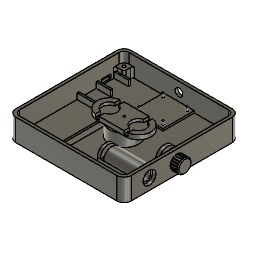
Microstir V2 (Autodesk Fusion 360 archive; units mm, degrees)
design "microstir" references "Type-C Lithium Battery Charger Board", "R300C DC Motor", "523450 Li-Ion Battery 3.7V 1000mAh", "PTFE Magnetic Stirrer Bar", "PWM DC motor speed controller", "Hexagon Socket Head Cap Screw STN EN ISO 4762 - M3 x 20 Steel 4.6 Plain"
Autodesk Fusion 360 part; units mm, degrees
(part 1 of 2)
sketch "Sketch1" plane through (0, 0, 0) normal (0, 0, 1) x (1, 0, 0)
  circle A0 centre (52.942, -52.6191) radius 1.6
  arc A1 (-47.558, -50.1191) -> (-49.558, -48.1191) centre (-49.558, -50.1191) ccw
  circle A2 centre (-52.058, -52.6191) radius 1.6
  line L0 (-49.558, -48.1191) -> (-54.558, -48.1191)
  arc A3 (-49.558, 47.8809) -> (-47.558, 49.8809) centre (-49.558, 49.8809) ccw
  line L1 (-56.558, -46.1191) -> (-56.558, 45.8809)
  line L2 (-59.558, -52.6191) -> (-59.558, 52.3809)
  arc A4 (-59.558, 52.3809) -> (-52.058, 59.8809) centre (-52.058, 52.3809) cw
  arc A5 (46.442, 56.8809) -> (48.442, 54.8809) centre (46.442, 54.8809) cw
  arc A6 (-45.558, -57.1191) -> (-47.558, -55.1191) centre (-45.558, -55.1191) cw
  line L3 (52.942, -60.1191) -> (-52.058, -60.1191)
  line L4 (-52.058, 59.8809) -> (52.942, 59.8809)
  arc A7 (-56.558, 45.8809) -> (-54.558, 47.8809) centre (-54.558, 45.8809) cw
  arc A8 (50.442, -48.1191) -> (48.442, -50.1191) centre (50.442, -50.1191) ccw
  arc A9 (48.442, 49.8809) -> (50.442, 47.8809) centre (50.442, 49.8809) ccw
  line L5 (48.442, 54.8809) -> (48.442, 49.8809)
  circle A10 centre (52.942, 52.3809) radius 1.6
  arc A11 (55.442, 47.8809) -> (57.442, 45.8809) centre (55.442, 45.8809) cw
  circle A12 centre (-52.058, 52.3809) radius 1.6
  arc A13 (-52.058, -60.1191) -> (-59.558, -52.6191) centre (-52.058, -52.6191) cw
  arc A14 (-47.558, 54.8809) -> (-45.558, 56.8809) centre (-45.558, 54.8809) cw
  line L6 (48.442, -50.1191) -> (48.442, -55.1191)
  arc A15 (-54.558, -48.1191) -> (-56.558, -46.1191) centre (-54.558, -46.1191) cw
  line L7 (57.442, 45.8809) -> (57.442, -46.1191)
  arc A16 (52.942, 59.8809) -> (60.442, 52.3809) centre (52.942, 52.3809) cw
  line L8 (50.442, 47.8809) -> (55.442, 47.8809)
  line L9 (-54.558, 47.8809) -> (-49.558, 47.8809)
  line L10 (55.442, -48.1191) -> (50.442, -48.1191)
  line L11 (60.442, 52.3809) -> (60.442, -52.6191)
  arc A17 (48.442, -55.1191) -> (46.442, -57.1191) centre (46.442, -55.1191) cw
  line L12 (-47.558, 49.8809) -> (-47.558, 54.8809)
  line L13 (-45.558, 56.8809) -> (46.442, 56.8809)
  line L14 (-47.558, -55.1191) -> (-47.558, -50.1191)
  arc A18 (57.442, -46.1191) -> (55.442, -48.1191) centre (55.442, -46.1191) cw
  arc A19 (60.442, -52.6191) -> (52.942, -60.1191) centre (52.942, -52.6191) cw
  line L15 (46.442, -57.1191) -> (-45.558, -57.1191)
  line L16 (-51.358, 56.8809) -> (52.242, 56.8809)
  line L17 (57.442, 51.6809) -> (57.442, -51.9191)
  line L18 (52.242, -57.1191) -> (-51.358, -57.1191)
  line L19 (-56.558, -51.9191) -> (-56.558, 51.6809)
  arc A20 (-51.358, 56.8809) -> (-56.558, 51.6809) centre (-51.358, 51.6809) ccw
  arc A21 (-56.558, -51.9191) -> (-51.358, -57.1191) centre (-51.358, -51.9191) ccw
  arc A22 (52.242, -57.1191) -> (57.442, -51.9191) centre (52.242, -51.9191) ccw
  arc A23 (57.442, 51.6809) -> (52.242, 56.8809) centre (52.242, 51.6809) ccw
  arc A24 (-79.7517, 57.5053) -> (-72.2517, 50.0053) centre (-79.7517, 50.0053) cw
  circle A25 centre (-79.7517, -54.9947) radius 1.6
  arc A26 (-184.7517, -62.4947) -> (-192.2517, -54.9947) centre (-184.7517, -54.9947) cw
  circle A27 centre (-184.7517, -54.9947) radius 1.6
  arc A28 (-72.2517, -54.9947) -> (-79.7517, -62.4947) centre (-79.7517, -54.9947) cw
  circle A29 centre (-184.7517, 50.0053) radius 1.6
  arc A30 (-192.2517, 50.0053) -> (-184.7517, 57.5053) centre (-184.7517, 50.0053) cw
  line L20 (-192.2517, -54.9947) -> (-192.2517, 50.0053)
  line L21 (-79.7517, -62.4947) -> (-184.7517, -62.4947)
  line L22 (-184.7517, 57.5053) -> (-79.7517, 57.5053)
  circle A31 centre (-79.7517, 50.0053) radius 1.6
  line L23 (-72.2517, 50.0053) -> (-72.2517, -54.9947)
  line L24 (-178.7517, 54.0053) -> (-85.7517, 54.0053)
  line L25 (-75.7517, 44.0053) -> (-75.7517, -48.9947)
  line L26 (-85.7517, -58.9947) -> (-178.7517, -58.9947)
  line L27 (-188.7517, -48.9947) -> (-188.7517, 44.0053)
  line L28 (-182.7517, -58.9947) -> (-184.2517, -58.9947)
  line L29 (-188.7517, -54.4947) -> (-188.7517, -52.9947)
  arc A32 (-80.2517, -58.9947) -> (-75.7517, -54.4947) centre (-80.2517, -54.4947) ccw
  arc A33 (-188.7517, -54.4947) -> (-184.2517, -58.9947) centre (-184.2517, -54.4947) ccw
  arc A34 (-184.2517, 54.0053) -> (-188.7517, 49.5053) centre (-184.2517, 49.5053) ccw
  line L30 (-132.2517, 54.0053) -> (-132.2517, -58.9947)
  line L31 (0.442, 56.8809) -> (0.442, -57.1191)
  line L32 (-75.7517, -52.9947) -> (-75.7517, -54.4947)
  line L33 (-81.7517, -58.9947) -> (-80.2517, -58.9947)
  line L34 (-75.7517, -48.9947) -> (-75.7517, -52.9947)
  line L35 (-85.7517, 54.0053) -> (-80.2517, 54.0053)
  line L36 (-184.2517, 54.0053) -> (-178.7517, 54.0053)
  line L37 (-188.7517, 44.0053) -> (-188.7517, 49.5053)
  line L38 (-188.7517, -48.9947) -> (-188.7517, -51)
  line L39 (-188.7517, -51) -> (-188.7517, -52.9947)
  line L40 (-178.7517, -58.9947) -> (-182.7517, -58.9947)
  line L41 (-85.7517, -58.9947) -> (-81.7517, -58.9947)
  line L42 (-74.6605, -54.9947) -> (-79.7517, -49.9035)
  line L43 (-79.7517, -49.9035) -> (-84.8428, -54.9947)
  line L44 (-84.8428, -54.9947) -> (-79.7517, -60.0858)
  line L45 (-79.7517, -60.0858) -> (-74.6605, -54.9947)
  line L46 (-74.6605, -54.9947) -> (-84.8428, -54.9947) construction
  line L47 (-79.7517, -49.9035) -> (-79.7517, -60.0858) construction
  line L48 (-84.8428, -54.9947) -> (-86.8428, -54.9947)
  line L49 (-86.8428, -54.9947) -> (-83.7517, -58.0858)
  line L50 (-79.7517, -49.9035) -> (-79.7517, -47.9035)
  line L51 (-79.7517, -47.9035) -> (-76.6605, -50.9947)
  line L52 (-76.6605, -50.9947) -> (-75.7517, -52.9947)
  line L53 (-83.7517, -58.0858) -> (-81.7517, -58.9947)
  line L54 (-79.7517, -47.9035) -> (-86.8428, -54.9947)
  line L55 (-79.7517, 44.9142) -> (-74.6605, 50.0053)
  line L56 (-74.6605, 50.0053) -> (-79.7517, 55.0965)
  line L57 (-79.7517, 55.0965) -> (-84.8428, 50.0053)
  line L58 (-84.8428, 50.0053) -> (-79.7517, 44.9142)
  line L59 (-84.8428, 50.0053) -> (-86.8428, 50.0053)
  line L60 (-86.8428, 50.0053) -> (-79.7517, 42.9142)
  line L61 (-86.8428, 50.0053) -> (-83.7517, 53.0965)
  line L62 (-83.7517, 53.0965) -> (-81.7517, 54.0053)
  line L63 (-81.7517, 54.0053) -> (-80.2517, 54.0053)
  line L64 (-75.7517, 48.0053) -> (-75.7517, 49.5053)
  arc A35 (-75.7517, 49.5053) -> (-80.2517, 54.0053) centre (-80.2517, 49.5053) ccw
  line L65 (-76.6605, 46.0053) -> (-75.7517, 48.0053)
  line L66 (-79.7517, 42.9142) -> (-76.6605, 46.0053)
  line L67 (-79.7517, 44.9142) -> (-79.7517, 42.9142)
  circle A36 centre (-79.7517, 50.0053) radius 1.6
  line L68 (-75.7517, 44.0053) -> (-75.7517, 48.7553)
  line L69 (-177.6605, -54.9947) -> (-184.7517, -47.9035)
  line L70 (-184.7517, -49.9035) -> (-184.7517, -47.9035)
  line L71 (-189.8428, -54.9947) -> (-184.7517, -60.0858)
  line L72 (-184.7517, -60.0858) -> (-179.6605, -54.9947)
  line L73 (-184.7517, -49.9035) -> (-189.8428, -54.9947)
  line L74 (-187.8428, -50.9947) -> (-188.7517, -52.9947)
  line L75 (-184.7517, -47.9035) -> (-187.8428, -50.9947)
  line L76 (-188.7517, -52.9947) -> (-188.7517, -54.4947)
  line L77 (-182.7517, -58.9947) -> (-184.2517, -58.9947)
  arc A37 (-188.7517, -54.4947) -> (-184.2517, -58.9947) centre (-184.2517, -54.4947) ccw
  line L78 (-180.7517, -58.0858) -> (-182.7517, -58.9947)
  line L79 (-177.6605, -54.9947) -> (-180.7517, -58.0858)
  line L80 (-179.6605, -54.9947) -> (-177.6605, -54.9947)
  line L81 (-179.6605, -54.9947) -> (-184.7517, -49.9035)
  circle A38 centre (-184.7517, -54.9947) radius 1.6
  line L82 (-184.7517, 42.9142) -> (-177.6605, 50.0053)
  line L83 (-184.7517, 44.9142) -> (-179.6605, 50.0053)
  line L84 (-184.7517, 55.0965) -> (-189.8428, 50.0053)
  line L85 (-189.8428, 50.0053) -> (-184.7517, 44.9142)
  line L86 (-179.6605, 50.0053) -> (-184.7517, 55.0965)
  line L87 (-179.6605, 50.0053) -> (-177.6605, 50.0053)
  line L88 (-180.7517, 53.0965) -> (-182.7517, 54.0053)
  line L89 (-182.7517, 54.0053) -> (-184.2517, 54.0053)
  arc A39 (-184.2517, 54.0053) -> (-188.7517, 49.5053) centre (-184.2517, 49.5053) ccw
  line L90 (-188.7517, 48.0053) -> (-188.7517, 49.5053)
  line L91 (-187.8428, 46.0053) -> (-188.7517, 48.0053)
  line L92 (-184.7517, 42.9142) -> (-187.8428, 46.0053)
  line L93 (-177.6605, 50.0053) -> (-180.7517, 53.0965)
  line L94 (-184.7517, 44.9142) -> (-184.7517, 42.9142)
  circle A40 centre (-184.7517, 50.0053) radius 1.6
  point P0 (52.942, -52.6191)
  point P1 (0.442, -0.1191)
  point P2 (-52.058, -52.6191)
  point P3 (-52.058, 52.3809)
  point P4 (52.942, 52.3809)
  point P5 (-79.7517, -54.9947)
  point P6 (-184.7517, -54.9947)
  point P7 (-184.7517, 50.0053)
  point P8 (-79.7517, 50.0053)
  point P9 (-132.2517, -2.4947)
  point P10 (-79.7517, -54.9947)
  point P11 (-79.7517, -54.9947)
  dimension "d1" = 5.2
  dimension "d195" = 7.2
  dimension "d196" = 7.2
  dimension "d199" = 2
  dimension "d202" = 2
  dimension "d203" = 7.2
  dimension "d204" = 7.2
  dimension "d205" = 2
  dimension "d206" = 2
  dimension "d207" = 7.2
  dimension "d208" = 7.2
  dimension "d209" = 2
  dimension "d210" = 2
  dimension "d211" = 7.2
  dimension "d212" = 7.2
  dimension "d213" = 2
  dimension "d214" = 2
  constraint horizontal L16
  constraint vertical L17
  constraint horizontal L18
  constraint vertical L19
  constraint tangent L16 A20
  constraint tangent L19 A20
  constraint tangent L18 A21
  constraint tangent L19 A21
  constraint equal A20 A21
  constraint tangent L17 A22
  constraint tangent L18 A22
  constraint equal A20 A22
  constraint tangent L16 A23
  constraint tangent L17 A23
  constraint equal A20 A23
  constraint horizontal L24
  constraint perpendicular L24 L25
  constraint parallel L24 L26
  constraint parallel L25 L27
  constraint coincident P11 P10
  constraint horizontal L28
  constraint vertical L29
  constraint tangent L28 A32
  constraint tangent L28 A33
  constraint tangent L29 A33
  constraint tangent L29 A34
  constraint midpoint L24 L30.start
  constraint midpoint L26 L30.end
  constraint midpoint L13 L31.start
  constraint midpoint L15 L31.end
  constraint coincident L28 A32.start
  constraint coincident L29 A34.end
  constraint coincident L25.end L32
  constraint coincident L26.start L33
  constraint perpendicular L42 L43
  constraint parallel L42 L44
  constraint parallel L43 L45
  constraint coincident L46 P11
  constraint coincident L47 P11
  constraint parallel L46 L48
  constraint vertical L50
  constraint perpendicular L49 L54
  constraint perpendicular L57 L58
  constraint parallel L55 L57
  constraint parallel L56 L58
  constraint perpendicular L60 L66
  constraint midpoint L64 L68.end
  constraint parallel L64 L68
  constraint perpendicular L72 L81
  constraint parallel L72 L73
  constraint parallel L71 L81
  constraint perpendicular L69 L75
  constraint perpendicular L83 L85
  constraint parallel L85 L86
  constraint parallel L83 L84
  constraint perpendicular L82 L93
  measures "d1" radius of A20
  measures "d195" distance of L43.end L44.end
  measures "d196" distance of L42.end L43.end
  measures "d199" distance of L43.end L48.end
  measures "d202" distance of L42.end L50.end
  measures "d203" distance of L55.end L55.start
  measures "d204" distance of L57.end L55.start
  measures "d205" distance of L55.start L60.end
  measures "d206" distance of L57.end L59.end
  measures "d207" distance of L71.start L70.start
  measures "d208" distance of L72.end L70.start
  measures "d209" distance of L70.start L69.end
  measures "d210" distance of L72.end L69.start
  measures "d211" distance of L84.start L83.end
  measures "d212" distance of L83.start L83.end
  measures "d213" distance of L82.end L83.end
  measures "d214" distance of L83.start L82.start
extrude "Extrude1" add sketch "Sketch1" along normal blind 2 contours A24 A26 A28 A30 L20 L21 L22 L23 | A25 | A27 A38 | A29 A40 | A31 A36 | L24 L26 L27 L30 L36 L37 L38 L39 L40 L69 L74 L75 L78 L79 L82 L88 L91 L92 L93 | L24 L25 L26 L30 L34 L35 L41 L49 L51 L52 L53 L54 L60 L61 L62 L65 L66 L68 | L36 L86 L87 L88 L89 L93 | A34 L36 L37 L83 L84 L85 L86 L89 A39 L90 | A34 L36 L84 L86 L89 A39 | L35 L57 L59 L61 L62 L63 | L82 L83 L87 L94 | L35 L56 L57 L63 A35 | L35 L55 L56 L57 L58 L63 L64 A35 | L33 L44 L48 L49 L53 | L28 L72 L77 L78 L79 L80 | A34 L84 A39 | L37 L85 L90 L91 L92 L94 | L58 L59 L60 L67 | A32 L32 L33 L42 L43 L44 L45 | A32 L33 L44 L45 | L28 A33 L71 L72 L77 A37 | L28 L29 A33 L71 L72 L73 L76 L77 A37 L81 | A34 L37 L84 L85 A39 L90 | L56 A35 | L55 L64 L65 L66 L67 L68 | L43 L48 L50 L54 | L69 L70 L80 L81 | L55 L56 L64 A35 | A32 L45 | L32 L42 L50 L51 L52 | A33 L71 A37 | L29 L70 L73 L74 L75 L76 | A32 L32 L42 L45 | L29 A33 L71 L73 L76 A37 makes body 1
extrude "Extrude2" add sketch "Sketch1" along normal blind 2.5 separate body contours A1 L0 A3 L1 A6 A7 A14 A15 L9 L12 L13 L14 L15 L16 L18 L19 L31 | A5 A8 A9 L5 A11 L6 L7 L8 L10 A17 L13 A18 L15 L16 L17 L18 L31 makes body 2
extrude "Extrude3" add sketch "Sketch1" along normal blind 23 contours L2 A4 L3 L4 A13 A16 L11 A19 bodies 2
extrude "Extrude20" add sketch "Sketch1" along normal blind 10 from surface at 2 contours L36 L86 L87 L88 L89 L93 | A34 L36 L37 L83 L84 L85 L86 L89 A39 L90 | L35 L57 L59 L61 L62 L63 | L82 L83 L87 L94 | L35 L55 L56 L57 L58 L63 L64 A35 | L33 L44 L48 L49 L53 | L28 L72 L77 L78 L79 L80 | A34 L84 A39 | L37 L85 L90 L91 L92 L94 | L58 L59 L60 L67 | A32 L32 L33 L42 L43 L44 L45 | L28 L29 A33 L71 L72 L73 L76 L77 A37 L81 | L56 A35 | L55 L64 L65 L66 L67 L68 | L43 L48 L50 L54 | L69 L70 L80 L81 | A32 L45 | L32 L42 L50 L51 L52 | A33 L71 A37 | L29 L70 L73 L74 L75 L76 bodies 1
extrude "Extrude21" add sketch "Sketch1" along normal blind 12.5 contours A1 L0 A6 A15 L14 L18 L19 A21 | A3 A7 A14 L9 L12 L16 L19 A20 | A8 L6 L10 A17 A18 L17 L18 A22 | A5 A9 L5 A11 L8 L16 L17 A23 bodies 2
sketch "Sketch12" plane through (0, 0, 12) normal (0, 0, 1) x (-1, 0, 0)
  line L0 (81.7517, 58.9947) -> (80.2517, 58.9947)
  arc A0 (80.2517, 58.9947) -> (75.7517, 54.4947) centre (80.2517, 54.4947) ccw
  line L1 (75.7517, 54.4947) -> (75.7517, 52.9947)
  circle A1 centre (79.7517, 54.9947) radius 3.1
  line L2 (79.7517, 59.3787) -> (79.7517, 50.6106) construction
  line L3 (84.1357, 54.9947) -> (75.3676, 54.9947) construction
  line L4 (79.7517, 49.9035) -> (84.8428, 54.9947)
  line L5 (84.8428, 54.9947) -> (79.7517, 60.0858)
  line L6 (79.7517, 60.0858) -> (74.6605, 54.9947)
  line L7 (74.6605, 54.9947) -> (79.7517, 49.9035)
  line L8 (79.7517, 49.9035) -> (79.7517, 60.0858) construction
  line L9 (84.8428, 54.9947) -> (74.6605, 54.9947) construction
  line L10 (79.7517, 60.0858) -> (74.6605, 60.0858)
  line L11 (74.6605, 60.0858) -> (74.6605, 54.9947)
  line L12 (74.6605, 54.9947) -> (79.7517, 54.9947)
  line L13 (79.7517, 54.9947) -> (79.7517, 60.0858)
  circle A2 centre (79.7517, 54.9947) radius 1.6
  line L14 (76.6605, 50.9947) -> (79.7517, 47.9035)
  line L15 (79.7517, 47.9035) -> (86.8428, 54.9947)
  line L16 (86.8428, 54.9947) -> (83.7517, 58.0858)
  line L17 (83.7517, 58.0858) -> (81.7517, 58.9947)
  line L18 (75.7517, 52.9947) -> (76.6605, 50.9947)
  line L19 (184.7517, 54.9947) -> (189.8428, 54.9947)
  line L20 (184.7517, 50.6106) -> (184.7517, 59.3787) construction
  circle A3 centre (184.7517, 54.9947) radius 3.1
  line L21 (189.8428, 60.0858) -> (184.7517, 60.0858)
  line L22 (179.6605, 54.9947) -> (184.7517, 49.9035)
  line L23 (184.7517, 49.9035) -> (189.8428, 54.9947)
  line L24 (184.7517, 49.9035) -> (184.7517, 60.0858) construction
  line L25 (189.8428, 54.9947) -> (189.8428, 60.0858)
  line L26 (184.7517, 60.0858) -> (179.6605, 54.9947)
  line L27 (189.8428, 54.9947) -> (184.7517, 60.0858)
  line L28 (189.1357, 54.9947) -> (180.3676, 54.9947) construction
  line L29 (179.6605, 54.9947) -> (189.8428, 54.9947) construction
  line L30 (184.7517, 60.0858) -> (184.7517, 54.9947)
  line L31 (79.7517, -55.0965) -> (79.7517, -50.0053)
  circle A4 centre (184.7517, -50.0053) radius 3.1
  line L32 (79.7517, -44.9142) -> (79.7517, -55.0965) construction
  line L33 (184.7517, -55.0965) -> (189.8428, -55.0965)
  line L34 (189.8428, -55.0965) -> (189.8428, -50.0053)
  line L35 (74.6605, -50.0053) -> (79.7517, -55.0965)
  line L36 (180.3676, -50.0053) -> (189.1357, -50.0053) construction
  line L37 (179.6605, -50.0053) -> (189.8428, -50.0053) construction
  line L38 (189.8428, -50.0053) -> (184.7517, -44.9142)
  line L39 (184.7517, -44.9142) -> (184.7517, -55.0965) construction
  line L40 (184.7517, -50.0053) -> (184.7517, -55.0965)
  line L41 (184.7517, -55.0965) -> (189.8428, -50.0053)
  line L42 (79.7517, -45.6213) -> (79.7517, -54.3894) construction
  line L43 (79.7517, -50.0053) -> (74.6605, -50.0053)
  line L44 (189.8428, -50.0053) -> (184.7517, -50.0053)
  line L45 (179.6605, -50.0053) -> (184.7517, -55.0965)
  line L46 (184.7517, -44.9142) -> (179.6605, -50.0053)
  circle A5 centre (79.7517, -50.0053) radius 3.1
  line L47 (79.7517, -55.0965) -> (84.8428, -50.0053)
  line L48 (84.8428, -50.0053) -> (74.6605, -50.0053) construction
  line L49 (74.6605, -50.0053) -> (74.6605, -55.0965)
  line L50 (75.3676, -50.0053) -> (84.1357, -50.0053) construction
  line L51 (74.6605, -55.0965) -> (79.7517, -55.0965)
  line L52 (84.8428, -50.0053) -> (79.7517, -44.9142)
  line L53 (79.7517, -44.9142) -> (74.6605, -50.0053)
  line L54 (184.7517, -54.3894) -> (184.7517, -45.6213) construction
  point P0 (79.7517, 54.9947)
  point P1 (79.7517, 54.9947)
  point P2 (184.7517, 54.9947)
  point P3 (184.7517, 54.9947)
  point P4 (79.7517, -50.0053)
  point P5 (79.7517, -50.0053)
  point P6 (184.7517, -50.0053)
  point P7 (184.7517, -50.0053)
  dimension "d184" = 6.2
  dimension "d190" = 7.2
  dimension "d191" = 7.2
  dimension "d215" = 6.2
  dimension "d216" = 7.2
  dimension "d217" = 7.2
  dimension "d218" = 6.2
  dimension "d219" = 7.2
  dimension "d220" = 7.2
  dimension "d221" = 6.2
  dimension "d222" = 7.2
  dimension "d223" = 7.2
  constraint coincident L2 P1
  constraint coincident L3 P1
  constraint coincident P1 P0
  constraint perpendicular L4 L5
  constraint parallel L4 L6
  constraint parallel L5 L7
  constraint coincident L8 P1
  constraint coincident L9 P1
  constraint horizontal L10
  constraint vertical L11
  constraint horizontal L12
  constraint vertical L13
  constraint coincident P3 L28
  constraint coincident P3 L20
  constraint coincident P3 P2
  constraint perpendicular L22 L23
  constraint parallel L22 L27
  constraint parallel L23 L26
  constraint coincident P3 L29
  constraint coincident P3 L24
  constraint coincident P5 L50
  constraint coincident P5 L42
  constraint coincident P5 P4
  constraint perpendicular L52 L53
  constraint parallel L35 L52
  constraint parallel L47 L53
  constraint coincident P5 L48
  constraint coincident P5 L32
  constraint coincident P7 L54
  constraint coincident P7 L36
  constraint coincident P7 P6
  constraint perpendicular L45 L46
  constraint parallel L41 L46
  constraint parallel L38 L45
  constraint coincident P7 L39
  constraint coincident P7 L37
  measures "d184" diameter of A1
  measures "d190" distance of L5.end L6.end
  measures "d191" distance of L4.end L5.end
  measures "d215" diameter of A3
  measures "d216" distance of L19.end L21.end
  measures "d217" distance of L19.end L22.end
  measures "d218" diameter of A5
  measures "d219" distance of L35.start L31.start
  measures "d220" distance of L35.start L32.start
  measures "d221" diameter of A4
  measures "d222" distance of L34.end L33.start
  measures "d223" distance of L33.start L37.start
extrude "Extrude34" cut sketch "Sketch12" against normal blind 3.5 from surface at -4 contours L0 A0 L1 A1 L4 L5 L7 L12 L13 | L0 A0 L5 L13 | A0 L6 L13 | A0 L6 L10 L11 | A0 A1 L6 L12 L13 | A0 L6 | A1 L12 L13 A2 | A1 L12 L13 A2 | A0 L1 L7 L12 | A0 L6 L12 | L12 L13 A2 | L12 L13 A2 | L19 A3 L30 | L19 A3 L30 | L19 A3 L27 L30 | L19 A3 L22 L23 L26 L30 | L21 L25 L27 | L31 L35 L43 A5 | L35 L49 L51 | L31 L43 A5 L47 L52 L53 | L31 L43 A5 | L31 L43 A5 | A4 L40 L44 | A4 L40 L41 L44 | A4 L38 L40 L44 L45 L46 | A4 L40 L44 | L33 L34 L41 bodies 1
fillet "Fillet1" radius 1 8 edges at (-79.7517, 42.9142, 7) (-86.8428, 50.0053, 7) (-177.6605, 50.0053, 7) (-184.7517, 42.9142, 7) (-184.7517, -47.9035, 7) (-177.6605, -54.9947, 7) (-86.8428, -54.9947, 7) (-79.7517, -47.9035, 7) on bodies 1
move_body "Move3" bodies 2 to x (1, 0, 0) y (0, 1, 0) z (0, 0, 1) at (77.465, -95.1704, 0)
move_body "Move4" bodies 2 to x (1, 0, 0) y (0, 1, 0) z (0, 0, 1) at (-77.9069, 95.2895, 0)
sketch "Sketch2" plane through (-60, 0, 0) normal (-1, 0, 0) x (0, -1, 0)
  line L0 (-52.5, 0) -> (52.5, 0)
  line L1 (52.5, 0) -> (52.5, 23)
  line L2 (52.5, 23) -> (-52.5, 23)
  line L3 (-52.5, 23) -> (-52.5, 0)
  line L4 (-33.8275, 8.1) -> (-33.3275, 8.1)
  line L5 (-43.325, 4.6) -> (-43.325, 4.1)
  line L6 (-42.825, 4.1) -> (-33.8275, 4.1)
  line L7 (-33.3275, 4.6) -> (-33.3275, 7.6)
  line L8 (-33.8275, 8.1) -> (-42.825, 8.1)
  line L9 (-43.325, 7.6) -> (-43.325, 4.6)
  line L10 (-42.825, 8.1) -> (-43.325, 7.6)
  line L11 (-33.8275, 8.1) -> (-33.3275, 7.6)
  line L12 (-33.8275, 4.1) -> (-33.3275, 4.6)
  line L13 (-43.325, 4.6) -> (-42.825, 4.1)
  point P0 (-33.3275, 4.1)
  point P1 (-43.325, 8.1)
  dimension "d27" = 0.5
  dimension "d29" = 0.5
  dimension "d30" = 0.5
  dimension "d31" = 0.5
  dimension "d32" = 0.5
  dimension "d33" = 0.5
  dimension "d34" = 0.5
  dimension "d35" = 0.5
  dimension "d36" = 0.5
  dimension "d37" = 0.5
  constraint horizontal L6
  constraint vertical L7
  constraint horizontal L8
  constraint vertical L9
  constraint coincident P1 L8
  constraint coincident P1 L9
  constraint coincident L4.end L8
  constraint coincident L4.end L7
  constraint coincident P0 L6
  constraint coincident P0 L7
  constraint coincident L5.end L9
  constraint coincident L5.end L6
  measures "d27" distance of L4.start L4.end
  measures "d29" distance of L5.start L5.end
  measures "d30" distance of P1 L8.end
  measures "d31" distance of P1 L9.start
  measures "d32" distance of L4.end L4.start
  measures "d33" distance of L4.end L7.end
  measures "d34" distance of P0 L6.end
  measures "d35" distance of P0 L7.start
  measures "d36" distance of L5.end L5.start
  measures "d37" distance of L5.end L6.start
extrude "Extrude6" cut sketch "Sketch2" against normal blind 3.5 contours L6 L7 L8 L9 L10 L11 L12 L13 bodies 2
sketch "Sketch3" plane through (0, 60, 0) normal (0, 1, 0) x (-1, 0, 0)
  line L0 (-52.5, 0) -> (52.5, 0)
  line L1 (52.5, 0) -> (52.5, 23)
  line L2 (52.5, 23) -> (-52.5, 23)
  line L3 (-52.5, 23) -> (-52.5, 0)
  line L4 (0, 20) -> (0, 6)
  circle A0 centre (0, 13) radius 4
  dimension "d40" = 8
  constraint vertical L4
  constraint midpoint L4 A0.centre
  measures "d40" diameter of A0
extrude "Extrude7" cut sketch "Sketch3" against normal blind 6 contours L4 A0 | L4 A0 bodies 2
sketch "Sketch4" plane through (57, 0, 0) normal (-1, 0, 0) x (0, -1, 0)
  line L0 (-46, 2.5) -> (46, 2.5)
  line L1 (51.8, 23) -> (-51.8, 23)
  line L2 (33.5, 15.45) -> (33.5, 7.5286)
  line L3 (29.64, 11.5) -> (37.3963, 11.5)
  circle A0 centre (33.5181, 11.5) radius 4.75
  circle A1 centre (33.5181, 11.5) radius 8.75
  line L4 (33.5181, 11.5) -> (24.7681, 11.5)
  line L5 (33.5181, 11.5) -> (42.2681, 11.5)
  line L6 (24.7681, 11.5) -> (24.7681, 2.5)
  line L7 (42.2681, 11.5) -> (42.2681, 2.5)
  line L8 (24.7681, 11.5) -> (24.7681, 2)
  line L9 (24.7681, 2) -> (42.2681, 2)
  line L10 (42.2681, 2) -> (42.2681, 11.5)
  line L11 (-46, 12.5) -> (-46, 2.5)
  line L12 (46, 2.5) -> (46, 12.5)
  line L13 (46, 12.5) -> (51.8, 12.5)
  line L14 (51.8, 12.5) -> (51.8, 23)
  line L15 (-51.8, 23) -> (-51.8, 12.5)
  line L16 (-51.8, 12.5) -> (-46, 12.5)
  dimension "d43" = 9.5
  dimension "d44" = 17.5
  constraint vertical L2
  constraint horizontal L3
  constraint midpoint L3 A0.centre
  constraint concentric A0 A1
  constraint coincident A0.centre A1.centre
  constraint coincident A1 L4.end
  constraint perpendicular L2 L4
  constraint coincident A1 L5.end
  constraint perpendicular L2 L5
  constraint coincident L0 L6.end
  constraint tangent A1 L6
  constraint coincident L0 L7.end
  constraint tangent A1 L7
  constraint tangent A1 L8
  constraint perpendicular L7 L9
  constraint tangent A1 L10
  measures "d43" diameter of A0
  measures "d44" diameter of A1
extrude "Extrude8" cut sketch "Sketch4" against normal blind 7 contours L3 A0 L4 L5 | L3 A0 L4 L5 bodies 2
extrude "Extrude9" add sketch "Sketch4" along normal blind 33 contours L0 A1 L6 L7 L8 L10 | A0 A1 L4 L5 | A0 A1 L4 L5 bodies 2
extrude "Extrude10" add sketch "Sketch4" along normal blind 3 from surface at 33 contours L0 A1 L6 L7 L8 L10 | A0 A1 L4 L5 | A0 A1 L4 L5 | L3 A0 L4 L5 | L3 A0 L4 L5 bodies 2
sketch "Sketch5" plane through (21, 0, 0) normal (-1, 0, 0) x (0, -1, 0)
  line L0 (24.7681, 11.5) -> (24.7681, 2.5)
  line L1 (24.7681, 2.5) -> (42.2681, 2.5)
  line L2 (42.2681, 2.5) -> (42.2681, 11.5)
  arc A0 (42.2681, 11.5) -> (24.7681, 11.5) centre (33.5181, 11.5) ccw
  line L3 (24.7681, 11.5) -> (42.2681, 11.5)
  circle A1 centre (33.5181, 11.5) radius 4.25
  dimension "d52" = 8.5
  constraint coincident L0.start A0.end
  constraint coincident L2.end A0.start
  measures "d52" diameter of A1
extrude "Extrude11" add sketch "Sketch5" along normal blind 3.5 contours L0 L1 L2 L3 A1 bodies 2
extrude "Extrude12" add sketch "Sketch5" along normal blind 3 from surface at 3.5 bodies 2
sketch "Sketch6" plane through (60, 0, 0) normal (1, 0, 0) x (0, 1, 0)
  circle A0 centre (-33.5181, 11.5) radius 4.75
  line L0 (-52.5, 0) -> (52.5, 0)
  line L1 (52.5, 0) -> (52.5, 23)
  line L2 (52.5, 23) -> (-52.5, 23)
  line L3 (-52.5, 23) -> (-52.5, 0)
  circle A1 centre (-33.5181, 11.5) radius 4.75
  line L4 (-33.5181, 16.25) -> (-33.5181, 6.75)
  line L5 (-38.2681, 11.5) -> (-28.7681, 11.5)
  circle A2 centre (-33.5181, 11.5) radius 6.75
  line L6 (-33.5181, 11.5) -> (-26.7681, 11.5)
  line L7 (-26.7681, 11.5) -> (-11.7681, 11.5)
  circle A3 centre (-5.0181, 11.5) radius 6.75
  circle A4 centre (-5.0181, 11.5) radius 9.25
  line L8 (-14.2681, 11.5) -> (-14.2681, 0)
  line L9 (4.2319, 11.5) -> (4.2319, 0)
  dimension "d58" = 13.5
  dimension "d132" = 15
  dimension "d133" = 13.5
  dimension "d134" = 18.5
  constraint tangent A0 A1
  constraint coincident A1 L4.start
  constraint coincident A0 L4.end
  constraint coincident A1 L5.start
  constraint coincident A1 L5.end
  constraint perpendicular L4 L5
  constraint concentric A0 A2
  constraint coincident A0.centre A1.centre
  constraint coincident A2 L6.end
  constraint perpendicular L4 L6
  constraint perpendicular L4 L7
  constraint coincident L7.end A3
  constraint concentric A3 A4
  constraint coincident A4 L8.start
  constraint coincident L7 L8.start
  constraint coincident L0 L8.end
  constraint tangent A4 L8
  constraint perpendicular L0 L8
  constraint coincident A4 L9.start
  constraint coincident L0 L9.end
  constraint tangent A4 L9
  constraint perpendicular L0 L9
  measures "d58" diameter of A2
  measures "d132" distance of L6.end L7.end
  measures "d133" diameter of A3
  measures "d134" diameter of A4
extrude "Extrude13" cut sketch "Sketch6" against normal blind 3.5 contours A2 bodies 2
sketch "Sketch8" plane through (0, 0, 0) normal (0, 0, 1) x (1, 0, 0)
  circle A0 centre (100, -50) radius 7.25
  circle A1 centre (100, -50) radius 6.5
  line L0 (100, -50) -> (100, -57.25)
  circle A2 centre (100, -57.25) radius 0.25
  line L1 (100, -50) -> (100, -42.4161)
  circle A3 centre (100, -50) radius 4.4
  dimension "d66" = 14.5
  dimension "d67" = 13
  dimension "d81" = 8.8
  constraint concentric A0 A1
  constraint coincident A0.centre A1.centre
  constraint coincident A0 L0.end
  constraint vertical L0
  constraint coincident L0.end A2.centre
  constraint parallel L0 L1
  constraint concentric A0 A3
  measures "d66" diameter of A0
  measures "d67" diameter of A1
  measures "d81" diameter of A3
extrude "Extrude15" add sketch "Sketch8" along normal blind 8 separate body contours A0 A1 L0 A2 L1 | A0 A1 L0 A2 L1 | A1 L0 L1 A3 | L0 L1 A3 picked at (103.5507, -54.5686) picked at (101.4022, -47.432) makes body 3
extrude "Extrude16" add sketch "Sketch8" along normal blind 3.5 from surface at 8 contours A1 L0 L1 A3 | L0 L1 A3 picked at (103.5507, -54.5686) picked at (101.4022, -47.432) bodies 3
extrude "Extrude17" add sketch "Sketch8" along normal blind 11.5 contours A1 L0 L1 A3 | L0 L1 A3 picked at (97.989, -44.576) picked at (97.8557, -48.0104) bodies 3
chamfer "Chamfer1" distance 1 angle 45 1 edges at (100, -42.75, 0) on bodies 3
pattern_circular "C-Pattern1" count 20 over 360 about axis through (100, -50, 8) along (0, 0, 1) of 1 faces at (100.2376, -57.1723, 3.2841) on bodies 3
extrude "Extrude18" cut sketch "Sketch8" along normal blind 3.5 from surface at 7.5 contours L0 L1 A3 | L0 L1 A3 bodies 3
sketch "Sketch9" plane through (0, 0, 2.5) normal (0, 0, 1) x (-1, 0, 0)
  line L0 (-14.5, 24.7681) -> (-57, 24.7681)
  line L1 (-57, 24.7681) -> (-57, -46)
  line L2 (-46, -57) -> (46, -57)
  line L3 (57, -46) -> (57, 46)
  line L4 (46, 57) -> (-46, 57)
  line L5 (-57, 42.2681) -> (-14.5, 42.2681)
  line L6 (-14.5, 42.2681) -> (-14.5, 24.7681)
  line L7 (25, 36) -> (23, 36)
  line L8 (40, 48) -> (32.323, 48)
  line L9 (40, 48) -> (48, 48)
  line L10 (23, 36) -> (23, 1)
  line L11 (23, 1) -> (23, 36)
  arc A0 (-57, -46) -> (-55, -48) centre (-55, -46) ccw
  line L12 (-55, -48) -> (-50, -48)
  arc A1 (-48, -50) -> (-50, -48) centre (-50, -50) ccw
  line L13 (-48, -50) -> (-48, -55)
  arc A2 (-48, -55) -> (-46, -57) centre (-46, -55) ccw
  arc A3 (46, -57) -> (48, -55) centre (46, -55) ccw
  line L14 (48, -55) -> (48, -50)
  arc A4 (50, -48) -> (48, -50) centre (50, -50) ccw
  line L15 (50, -48) -> (55, -48)
  arc A5 (55, -48) -> (57, -46) centre (55, -46) ccw
  arc A6 (57, 46) -> (55, 48) centre (55, 46) ccw
  line L16 (55, 48) -> (50, 48)
  arc A7 (48, 50) -> (50, 48) centre (50, 50) ccw
  line L17 (48, 50) -> (48, 55)
  arc A8 (48, 55) -> (46, 57) centre (46, 55) ccw
  arc A9 (-46, 57) -> (-48, 55) centre (-46, 55) ccw
  line L18 (-48, 55) -> (-48, 50)
  arc A10 (-50, 48) -> (-48, 50) centre (-50, 50) ccw
  line L19 (-50, 48) -> (-55, 48)
  arc A11 (-55, 48) -> (-57, 46) centre (-55, 46) ccw
  line L20 (-57, 46) -> (-57, 42.2681)
  line L21 (54, -31) -> (54, -30)
  line L22 (53.2755, -45.4626) -> (53.2755, -46.4626)
  line L23 (57, -30) -> (42, -30)
  line L24 (42, -30) -> (42, -28)
  line L25 (42, -28) -> (57, -28)
  line L26 (57, -28) -> (57, -30)
  line L27 (56.9458, -46.4626) -> (41.9458, -46.4626)
  line L28 (41.9458, -46.4626) -> (41.9458, -48.4626)
  line L29 (41.9458, -48.4626) -> (56.9458, -48.4626)
  line L30 (56.9458, -48.4626) -> (56.9458, -46.4626)
  line L31 (0, -12.25) -> (0, 12.25)
  circle A12 centre (0, 0) radius 12.15
  line L32 (-5, -13.25) -> (-5, -11)
  circle A13 centre (0, 0) radius 15.15
  line L33 (5, -11) -> (-5, -11)
  line L34 (-5, -11) -> (-5, -16)
  line L35 (-5, -16) -> (5, -16)
  line L36 (5, -16) -> (5, -11)
  line L37 (16, -24.5) -> (-16, -24.5)
  line L38 (-16, -24.5) -> (-16, -57)
  line L39 (-16, -57) -> (16, -57)
  line L40 (16, -57) -> (16, -24.5)
  circle A14 centre (-12.5, -28) radius 1
  circle A15 centre (12.5, -28) radius 1
  circle A16 centre (12.5, -53) radius 1
  circle A17 centre (-12.5, -53) radius 1
  line L41 (57, -6.1113) -> (23.05, -6.1113)
  line L42 (23.05, -6.1113) -> (23.05, 45.89)
  line L43 (23.05, 45.89) -> (57, 45.89)
  line L44 (57, 45.89) -> (57, -6.1113)
  line L45 (23.05, 44.6006) -> (23.05, 42.7046)
  line L46 (23.05, -6.1113) -> (26.55, -6.1113)
  line L47 (23.05, -6.1113) -> (23.05, -4.1113)
  line L48 (23.05, -4.1113) -> (21.05, -4.1113)
  line L49 (21.05, -4.1113) -> (21.05, -6.5055)
  line L50 (21.05, -6.5055) -> (23.05, -6.5055)
  line L51 (23.05, -6.5055) -> (23.05, -4.1113)
  line L52 (26.55, -6.1113) -> (23.5988, -6.1113)
  line L53 (23.5988, -6.1113) -> (23.5988, -8.1113)
  line L54 (23.5988, -8.1113) -> (26.55, -8.1113)
  line L55 (26.55, -8.1113) -> (26.55, -6.1113)
  line L56 (26.55, -8.1113) -> (57, -8.1113)
  line L57 (57, -8.1113) -> (57, -10.1113)
  line L58 (57, -10.1113) -> (26.55, -10.1113)
  line L59 (26.55, -10.1113) -> (26.55, -8.1113)
  line L60 (23.05, 45.89) -> (21.05, 45.89)
  line L61 (21.05, 45.89) -> (21.05, 47.89)
  line L62 (21.05, 47.89) -> (23.05, 47.89)
  line L63 (23.05, 47.89) -> (23.05, 45.89)
  line L64 (21.05, 47.89) -> (57.8185, 47.89)
  line L65 (57.8185, 47.89) -> (57.8185, 49.89)
  line L66 (57.8185, 49.89) -> (21.05, 49.89)
  line L67 (21.05, 49.89) -> (21.05, 47.89)
  line L68 (21.05, 49.89) -> (20.05, 49.89)
  line L69 (19.05, 48.89) -> (19.05, -6.511)
  line L70 (19.05, -6.511) -> (21.05, -6.511)
  line L71 (21.05, -6.511) -> (21.05, 49.89)
  arc A18 (20.05, 49.89) -> (19.05, 48.89) centre (20.05, 48.89) ccw
  line L72 (21.05, -4.1113) -> (19.05, -4.1113)
  point P0 (0, -12.15)
  point P1 (19.05, -10.1113)
  point P2 (19.05, 49.89)
  dimension "d98" = 1
  dimension "d99" = 1
  dimension "d100" = 15
  dimension "d101" = 2
  dimension "d104" = 24.5
  dimension "d105" = 24.3
  dimension "d107" = 30.3
  dimension "d110" = 2
  dimension "d111" = 2
  dimension "d112" = 2
  dimension "d113" = 2
  dimension "d174" = 3.5
  dimension "d175" = 2
  dimension "d176" = 2
  dimension "d177" = 2
  dimension "d178" = 2
  dimension "d179" = 2
  dimension "d180" = 2
  dimension "d181" = 2
  dimension "d182" = 2
  dimension "d183" = 1
  constraint horizontal L7
  constraint parallel L8 L9
  constraint perpendicular L7 L10
  constraint vertical L21
  constraint vertical L22
  constraint horizontal L23
  constraint vertical L24
  constraint horizontal L25
  constraint vertical L26
  constraint coincident L3 L23.start
  constraint horizontal L27
  constraint vertical L28
  constraint horizontal L29
  constraint vertical L30
  constraint coincident A5 L27.start
  constraint vertical L31
  constraint coincident A12.centre A13.centre
  constraint coincident A12 P0
  constraint vertical L32
  constraint concentric A12 A13
  constraint horizontal L33
  constraint vertical L34
  constraint horizontal L35
  constraint vertical L36
  constraint horizontal L37
  constraint vertical L38
  constraint horizontal L39
  constraint vertical L40
  constraint coincident L2 L38.end
  constraint horizontal L41
  constraint vertical L42
  constraint horizontal L43
  constraint vertical L44
  constraint coincident L3 L41.start
  constraint coincident L42 L45.start
  constraint coincident L42 L45.end
  constraint perpendicular L42 L46
  constraint perpendicular L46 L47
  constraint horizontal L48
  constraint vertical L49
  constraint horizontal L50
  constraint vertical L51
  constraint horizontal L52
  constraint vertical L53
  constraint horizontal L54
  constraint vertical L55
  constraint horizontal L56
  constraint vertical L57
  constraint horizontal L58
  constraint vertical L59
  constraint horizontal L60
  constraint vertical L61
  constraint horizontal L62
  constraint vertical L63
  constraint horizontal L64
  constraint vertical L65
  constraint horizontal L66
  constraint vertical L67
  constraint horizontal L68
  constraint vertical L69
  constraint horizontal L70
  constraint vertical L71
  constraint coincident P2 L68
  constraint coincident P2 L69
  constraint tangent L68 A18
  constraint tangent L69 A18
  constraint coincident L69 L72.end
  constraint perpendicular L69 L72
  measures "d98" distance of L21.start L21.end
  measures "d99" distance of L22.start L22.end
  measures "d100" distance of L27.start L27.end
  measures "d101" distance of L27.start L29.end
  measures "d104" distance of L31.start L31.end
  measures "d105" diameter of A12
  measures "d107" diameter of A13
  measures "d110" diameter of A14
  measures "d111" diameter of A15
  measures "d112" diameter of A16
  measures "d113" diameter of A17
  measures "d174" distance of L41.end L46.end
  measures "d175" distance of L41.end L47.end
  measures "d176" distance of L47.end L48.end
  measures "d177" distance of L46.end L54.end
  measures "d178" distance of L54.end L58.end
  measures "d179" distance of L42.end L60.end
  measures "d180" distance of L42.end L62.end
  measures "d181" distance of L61.end L66.end
  measures "d182" distance of L66.end P2
  measures "d183" radius of A18
extrude "Extrude19" add sketch "Sketch9" along normal blind 6 contours A6 L16 A7 L62 L64 L66 L67 L71 | L3 L56 L57 L58 L59 bodies 2
extrude "Extrude22" add sketch "Sketch9" along normal blind 6 contours A6 L16 A7 L62 L64 L66 L67 L71 | A4 L15 A5 L27 L28 L29 | L61 L67 L68 L69 L71 A18 L72 | L3 L23 L24 L25 L26 | L3 L56 L57 L58 L59 bodies 2
extrude "Extrude23" add sketch "Sketch9" along normal blind 13 contours A12 L32 A13 L34 L36 picked at (-12.8257, -5.9132) bodies 2
extrude "Extrude24" add sketch "Sketch9" along normal blind 2 contours L2 L37 L38 L39 L40 bodies 2
extrude "Extrude25" add sketch "Sketch9" along normal blind 6 contours A14 | A15 | A16 | A17 bodies 2
move_body "Move5" bodies 1 to x (1, 0, 0) y (0, 1, 0) z (0, 0, 1) at (132.2517, 2.4947, 0.5)
move_body "Move6" bodies 1 to x (-1, 0, 0) y (0, 1, 0) z (0, 0, -1) at (-120, 0, 1)
move_body "Move7" bodies 1 to x (1, 0, 0) y (0, 1, 0) z (0, 0, 1) at (120, 0, 2)
move_body "Move8" bodies 1 to x (1, 0, 0) y (0, 1, 0) z (0, 0, 1) at (0, 0, 22.5)
ref_plane "WorkPlane4" through (0, 0, 17) normal (0, 0, 1) x (1, 0, 0)
sketch "Sketch10" plane through (0, 0, 17) normal (0, 0, 1) x (1, 0, 0)
  line L0 (0.0002, 14.9991) -> (0.0002, -15.0009)
  circle A0 centre (0.0002, 14.9991) radius 7.75
  circle A1 centre (0.0002, -15.0009) radius 7.75
  circle A2 centre (0, 0) radius 1.15
  circle A3 centre (0.0002, 14.9991) radius 13
  circle A4 centre (0.0002, -15.0009) radius 13
  line L1 (0.0002, -15.0009) -> (13.0002, -15.0009)
  line L2 (0.0002, 14.9991) -> (13.0002, 14.9991)
  line L3 (13.0002, 14.9991) -> (13.0002, -15.0009)
  line L4 (-12.9998, 15.0006) -> (-12.9998, -15.0009)
  line L5 (0.0002, -22.7509) -> (0.0002, -28.0009)
  line L6 (7.7502, -15.0009) -> (13.0002, -15.0009)
  line L7 (-7.7498, -15.0009) -> (-12.9998, -15.0009)
  line L8 (-5.8781, -17.0083) -> (-14.8715, -17.0083)
  line L9 (-14.8715, -17.0083) -> (-14.8715, -12.9936)
  line L10 (-14.8715, -12.9936) -> (-5.8781, -12.9936)
  line L11 (-5.8781, -12.9936) -> (-5.8781, -17.0083)
  line L12 (-5.8781, -17.0083) -> (-14.8715, -12.9936) construction
  line L13 (-14.8715, -17.0083) -> (-5.8781, -12.9936) construction
  line L14 (6.3788, -17.0082) -> (14.3716, -17.0082)
  line L15 (14.3716, -17.0082) -> (14.3716, -12.9937)
  line L16 (14.3716, -12.9937) -> (6.3788, -12.9937)
  line L17 (6.3788, -12.9937) -> (6.3788, -17.0082)
  line L18 (6.3788, -17.0082) -> (14.3716, -12.9937) construction
  line L19 (14.3716, -17.0082) -> (6.3788, -12.9937) construction
  line L20 (-7.7498, 15.0006) -> (-12.9998, 15.0006)
  line L21 (7.7502, 14.9991) -> (13.0002, 14.9991)
  line L22 (-5.8781, 12.9932) -> (-14.8715, 12.9932)
  line L23 (-14.8715, 12.9932) -> (-14.8715, 17.0079)
  line L24 (-14.8715, 17.0079) -> (-5.8781, 17.0079)
  line L25 (-5.8781, 17.0079) -> (-5.8781, 12.9932)
  line L26 (-5.8781, 12.9932) -> (-14.8715, 17.0079) construction
  line L27 (-14.8715, 12.9932) -> (-5.8781, 17.0079) construction
  line L28 (14.8759, 13.0007) -> (5.8745, 13.0007)
  line L29 (5.8745, 13.0007) -> (5.8745, 16.9974)
  line L30 (5.8745, 16.9974) -> (14.8759, 16.9974)
  line L31 (14.8759, 16.9974) -> (14.8759, 13.0007)
  line L32 (14.8759, 13.0007) -> (5.8745, 16.9974) construction
  line L33 (5.8745, 13.0007) -> (14.8759, 16.9974) construction
  point P0 (0.0002, -0.0009)
  point P1 (-10.3748, -15.0009)
  point P2 (10.3752, -15.0009)
  point P3 (-10.3748, 15.0006)
  point P4 (10.3752, 14.9991)
  dimension "d119" = 30
  dimension "d120" = 15.5
  dimension "d121" = 15.5
  dimension "d122" = 2.3
  dimension "d123" = 26
  dimension "d124" = 26
  constraint midpoint L0 P0
  constraint vertical L0
  constraint coincident L0.start A0.centre
  constraint coincident L0.end A1.centre
  constraint coincident A2.centre origin
  constraint concentric A0 A3
  constraint concentric A1 A4
  constraint coincident A4 L1.end
  constraint perpendicular L0 L1
  constraint coincident A3 L2.end
  constraint perpendicular L0 L2
  constraint coincident A3 L4.start
  constraint coincident A4 L4.end
  constraint tangent A4 L4
  constraint coincident A1 L5.start
  constraint coincident A4 L5.end
  constraint vertical L5
  constraint coincident A1 L6.start
  constraint coincident L1 L6.start
  constraint coincident A1 L7.start
  constraint perpendicular L4 L7
  constraint horizontal L8
  constraint perpendicular L8 L9
  constraint parallel L8 L10
  constraint parallel L9 L11
  constraint coincident L12 P1
  constraint coincident L13 P1
  constraint midpoint L7 P1
  constraint horizontal L14
  constraint perpendicular L14 L15
  constraint parallel L14 L16
  constraint parallel L15 L17
  constraint coincident L18 P2
  constraint coincident L19 P2
  constraint midpoint L6 P2
  constraint coincident A0 L20.start
  constraint perpendicular L4 L20
  constraint coincident A0 L21.start
  constraint coincident L2 L21.start
  constraint horizontal L22
  constraint perpendicular L22 L23
  constraint parallel L22 L24
  constraint parallel L23 L25
  constraint coincident L26 P3
  constraint coincident L27 P3
  constraint midpoint L20 P3
  constraint horizontal L28
  constraint perpendicular L28 L29
  constraint parallel L28 L30
  constraint parallel L29 L31
  constraint coincident L32 P4
  constraint coincident L33 P4
  constraint midpoint L21 P4
  measures "d119" distance of L0.start L0.end
  measures "d120" diameter of A0
  measures "d121" diameter of A1
  measures "d122" diameter of A2
  measures "d123" diameter of A3
  measures "d124" diameter of A4
extrude "Extrude26" add sketch "Sketch10" against normal blind 1.5 separate body contours L0 A0 L2 L28 L29 | L0 A0 L2 L22 L24 L25 L29 L30 | L0 A0 A3 L28 | L0 A0 A3 L22 | A0 L2 L29 L30 | A0 L2 L28 L29 | L0 A2 A3 A4 L3 L16 L28 | L0 A2 A3 A4 L4 L10 L22 | A3 L4 L22 | A0 A3 L20 L22 | A0 L22 L24 L25 | A0 A3 L2 L21 L28 | A0 A3 L2 L21 L30 | A3 L3 L28 | A0 A3 L20 L24 | A0 A3 L24 L30 | L0 A1 A4 L16 | L0 A1 A4 L10 | A4 L4 L10 | A4 L3 L16 | L0 A1 L1 L16 L17 | L0 A1 L1 L8 L10 L11 L14 L17 | A1 A4 L1 L6 L16 | A1 A4 L7 L10 | A1 A4 L7 L8 | A1 A4 L1 L6 L14 | A1 L1 L16 L17 | A1 L8 L10 L11 | A1 A4 L5 L8 | A1 A4 L5 L14 | A1 L1 L14 L17 makes body 4
extrude "Extrude27" add sketch "Sketch10" along normal blind 3 contours L0 A0 A3 L28 | L0 A0 A3 L22 | L0 A2 A3 A4 L3 L16 L28 | L0 A2 A3 A4 L4 L10 L22 | A3 L4 L22 | A0 A3 L20 L22 | A0 A3 L2 L21 L28 | A0 A3 L2 L21 L30 | A3 L3 L28 | A0 A3 L20 L24 | A0 A3 L24 L30 | L0 A1 A4 L16 | L0 A1 A4 L10 | A4 L4 L10 | A4 L3 L16 | A1 A4 L1 L6 L16 | A1 A4 L7 L10 | A1 A4 L7 L8 | A1 A4 L1 L6 L14 | A1 A4 L5 L8 | A1 A4 L5 L14 bodies 4
extrude "Extrude28" cut sketch "Sketch10" along normal blind 4 contours A0 L2 L29 L30 | A0 L2 L28 L29 | A3 L4 L22 | A0 A3 L20 L22 | A0 L22 L24 L25 | A0 A3 L2 L21 L28 | A0 A3 L2 L21 L30 | A3 L3 L28 | A0 A3 L20 L24 | A3 L3 L28 L30 L31 | A3 L4 L22 L23 L24 | A4 L4 L10 | A4 L4 L8 L9 L10 | A4 L3 L14 L15 L16 | A4 L3 L16 | A1 A4 L1 L6 L16 | A1 A4 L7 L10 | A1 A4 L7 L8 | A1 A4 L1 L6 L14 | A1 L1 L16 L17 | A1 L8 L10 L11 | A1 L1 L14 L17 bodies 4
move_body "Move9" bodies 4 to x (0, -1, 0) y (1, 0, 0) z (0, 0, 1) at (0, 0, 0)
extrude "Extrude29" add sketch "Sketch6" against normal blind 6 contours L0 A4 L8 L9 | A4 | A3 bodies 2
extrude "Extrude30" cut sketch "Sketch6" against normal blind 3.5 contours A3 bodies 2
sketch "Sketch11" plane through (54, 0, 0) normal (-1, 0, 0) x (0, -1, 0)
  line L0 (-4.2319, 2.5) -> (14.2681, 2.5)
  line L1 (14.2681, 2.5) -> (14.2681, 11.5)
  arc A0 (14.2681, 11.5) -> (-4.2319, 11.5) centre (5.0181, 11.5) ccw
  line L2 (-4.2319, 11.5) -> (-4.2319, 2.5)
  line L3 (-4.2319, 11.5) -> (14.2681, 11.5)
  line L4 (5.0181, 20.75) -> (5.0181, 2.5)
  circle A1 centre (5.0181, 11.5) radius 4.25
  dimension "d140" = 8.5
  constraint coincident A0.end L2.start
  constraint coincident L1.end A0.start
  constraint midpoint A0 L4.start
  constraint midpoint L0 L4.end
  constraint concentric A0 A1
  measures "d140" diameter of A1
extrude "Extrude31" add sketch "Sketch11" along normal blind 3.5 contours L0 L2 L3 L4 A1 | L0 L1 L3 L4 A1 bodies 2
extrude "Extrude32" add sketch "Sketch11" along normal blind 3.5 from surface at 3.5 bodies 2
move_body "Move10" bodies 3 to x (1, 0, 0) y (0, 1, 0) z (0, 0, 1) at (-43.5, 44.9819, 0)
move_body "Move11" bodies 3 to x (0, 0, 1) y (0, 1, 0) z (-1, 0, 0) at (82.7533, 0, -49.2533)
move_body "Move12" bodies 3 to x (1, 0, 0) y (0, 1, 0) z (0, 0, 1) at (-14.7533, 0, 4.2533)
move_body "Move13" bodies 3 to x (1, 0, 0) y (0, 1, 0) z (0, 0, 1) at (0.2, 0, 0)
other "Screw1"
other "Screw2"
other "Screw3"
other "Screw4"
hidden bodies 1
equation "d35 = d34"
equation "d37 = d36"
equation "d44 = 9.500 mm + 8 mm"
equation "d58 = 9.500 mm + 4 mm"
equation "d96 = 23.00 mm - 10.5 mm"
equation "d107 = d105 + 6 mm"
equation "d120 = d121"
equation "d123 = 16.000 mm + 10 mm"
equation "d124 = 16.000 mm + 10 mm"
equation "d134 = 13.500 mm + 5 mm"
equation "d136 = -3.5 mm - 2.5 mm"

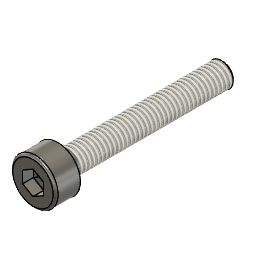
design "Hexagon Socket Head Cap Screw STN EN ISO 4762 - M3 x 20 Steel 4.6 Plain"
description: Hexagon Socket Head Cap Screw STN EN ISO 4762 - M3 x 20
part number: STN EN ISO 4762 - M3 x 20 Steel 4.6 Plain
Autodesk Fusion 360 part; units mm, degrees
sketch "Sketch1" plane through (0, 0, 0) normal (0, 1, 0) x (1, 0, 0)
  line L0 (-1.5, 0) -> (-1.5, 20)
  line L1 (-1.5, 20) -> (0, 20)
  line L2 (0, 20) -> (0, -3)
  line L3 (-1.5, 0) -> (-2.75, 0)
  line L4 (-2.75, 0) -> (-2.75, -3)
  line L5 (-2.75, -3) -> (0, -3)
  dimension "d9" = 3
  dimension "d106" = 3
  dimension "d107" = 20
  dimension "d116" = 5.5
  constraint perpendicular L0 L1
  constraint collinear origin L1.end L2.end
  constraint perpendicular L0 L3
  constraint coincident origin L3
  constraint vertical L2
  constraint coincident L2 L5.end
  constraint perpendicular L2 L5
  measures "d106" distance of L3 L5
  measures "d107" distance of origin L1
revolve "Revolve1" add sketch "Sketch1" angle 360 about axis through (0, 0, -20) along (0, 0, 1)
ref_plane "WorkPlane1" through (0, 0, 3) normal (0, 0, 1) x (1, 0, 0)
sketch "Sketch6" plane through (0, 0, 3) normal (0, 0, 1) x (1, 0, 0)
  line L0 (-1.25, 0.7217) -> (-1.25, -0.7217)
  line L1 (-1.25, -0.7217) -> (0, -1.4434)
  line L2 (0, -1.4434) -> (1.25, -0.7217)
  line L3 (1.25, -0.7217) -> (1.25, 0.7217)
  line L4 (1.25, 0.7217) -> (0, 1.4434)
  line L5 (0, 1.4434) -> (-1.25, 0.7217)
  dimension "d117" = 2.5
  constraint vertical L0
  measures "d117" distance of L0 L3
extrude "Extrude1" cut sketch "Sketch6" against normal blind 1.3
extrude "Extrude2" cut 1 faces at (-0.4167, 0.2406, 1.7) along direction (0, 0, -1) blind 1.3 draft -85
fillet "Fillet4" radius 0.3 1 edges at (-2.5639, 0.9944, 3)
thread "Thread3" "ISO Metric profile 3.0 M3x0.5 M3x0.5 6g" major diameter 2.927 minor diameter 2.3555 pitch 0.5 angle 60 resizes the face on face at (-1.4925, 0.1494, -13.3333) from (0, 0, -1.25) to (0, 0, -20)
sketch "Sketch7" plane through (0, 0, 0) normal (0, 1, 0) x (1, 0, 0)
  line L0 (-1.53, 20) -> (-1.53, 19.7)
  line L1 (-1.53, 19.7) -> (-1.23, 20)
  line L2 (0, 20) -> (0, -3)
  line L3 (-1.53, 20) -> (0, 20)
  dimension "d101" = 45
  dimension "d112" = 0.3
  dimension "d113" = 1.53
  constraint coincident L2.start L3.end
  constraint perpendicular L2 L3
  constraint coincident L1.end L3
  constraint perpendicular L0 L3
  measures "d101" angle of L0 L1
  measures "d112" distance of L0.end L3
  measures "d113" distance of L0 L2.start
revolve "Revolve3" cut sketch "Sketch7" angle 360 about axis through (0, 0, 1.75) along (0, 0, 1)
equation "d9 = adsk_nomdia"
equation "adsk_nomlen = 20.00 mm"
equation "adsk_headh = 3.00 mm"
equation "adsk_headdia = 5.50 mm"
equation "adsk_nomdia = 3.00 mm"
equation "adsk_philwidth = 2.50 mm"
equation "d31 = -adsk_phildepth"
equation "adsk_phildepth = 1.30 mm"
equation "d71 = adsk_headh"
equation "d76 = -adsk_phildepth"
equation "adsk_thrlen = 18.75 mm"
equation "d86 = adsk_nomdia * 0.1"
equation "adsk_startang = 45.00 deg"
equation "d101 = adsk_startang"
equation "adsk_pitch1 = 0.50 mm"
equation "adsk_startlen = 0.30 mm"
equation "d106 = adsk_headh"
equation "d107 = adsk_nomlen"
equation "d112 = adsk_startlen"
equation "d113 = adsk_nomdia * 0.51"
equation "d115 = min(adsk_thrlen; adsk_nomlen - 0.001 mm)"
equation "d116 = adsk_headdia"
equation "d117 = adsk_philwidth"

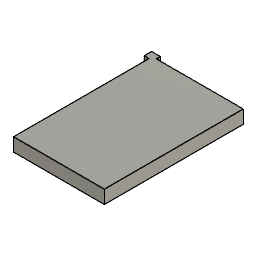
design "523450 Li-Ion Battery 3.7V 1000mAh"
Autodesk Fusion 360 part; units mm, degrees